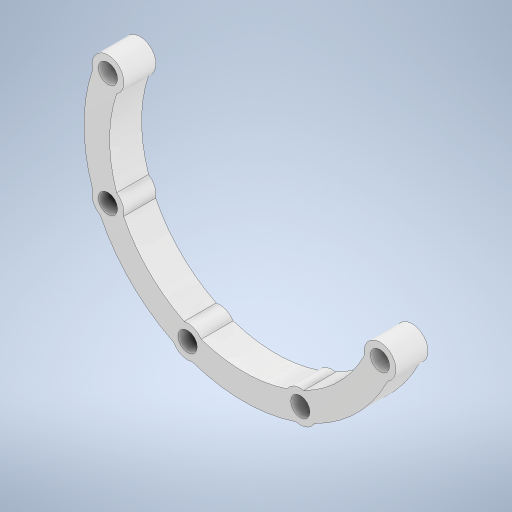
# Autodesk Inventor part: RP_Hip-Link-Limit-Long
Saved by Autodesk Inventor 2024.3 (Build 283343000, 343)
## iProperties
Created: 2025-01-05
Part Number: RP_Hip-Link-Limit-Long
Material: ABS プラスチック
Document SubType Name: Modeling
Designer: 佐藤智貴
Density: 1.06 g/cm^3
Appearance: 滑らか - 白
Mass: 12.4711 g
Surface Area: 64.1579 cm^2
Volume: 11.7652 cm^3
Author: 佐藤智貴
Autodesk Inventor part; units mm, degrees
ref_plane "YZ Plane" through (0, 0, 0) normal (1, 0, 0) x (0, 1, 0)
ref_plane "XZ Plane" through (0, 0, 0) normal (0, 1, 0) x (-1, 0, 0)
ref_plane "XY Plane" through (0, 0, 0) normal (0, 0, 1) x (1, 0, 0)
sketch "スケッチ1" plane through (0, 0, 0) normal (0, 0, 1) x (1, 0, 0)
  arc A0 (-41.8605, 19.0708) -> (-40.3368, 22.112) centre (0, 0) ccw
  line L0 (0, 0) -> (0, 54.8528)
  line L1 (0, 0) -> (-20.7697, 50.1426)
  circle A1 centre (-17.6034, 42.4985) radius 1.6
  circle A2 centre (-42.4985, 17.6034) radius 1.6
  circle A3 centre (-42.4985, -17.6034) radius 1.6
  circle A4 centre (-17.6034, -42.4985) radius 1.6
  circle A5 centre (17.6034, -42.4985) radius 1.6
  circle A6 centre (42.4985, -17.6034) radius 1.6
  circle A7 centre (42.4985, 17.6034) radius 1.6
  circle A8 centre (17.6034, 42.4985) radius 1.6
  line L2 (0, 0) -> (-55.1659, -46.2897)
  line L3 (-55.1659, -46.2897) -> (-55.1659, 46.2897)
  line L4 (-55.1659, 46.2897) -> (0, 0)
  line L5 (0, 0) -> (-76.7662, 0)
  circle A9 centre (-42.4985, 17.6034) radius 5
  circle A10 centre (-42.4985, -17.6034) radius 5
  circle A11 centre (-17.6034, -42.4985) radius 5
  circle A12 centre (17.6034, -42.4985) radius 5
  line L6 (0, 0) -> (55.1659, -46.2897)
  line L7 (55.1659, 46.2897) -> (0, 0)
  circle A13 centre (-17.6034, 42.4985) radius 5
  circle A14 centre (42.4985, -17.6034) radius 5
  arc A15 (-39.8089, 13.3884) -> (-39.8089, -13.3884) centre (0, 0) ccw
  arc A16 (-47.2999, 16.2085) -> (-47.2999, -16.2085) centre (0, 0) ccw
  arc A17 (-37.6162, -18.6821) -> (-18.6821, -37.6162) centre (0, 0) ccw
  arc A18 (-44.9073, -21.985) -> (-21.985, -44.9073) centre (0, 0) ccw
  arc A19 (-13.3884, -39.8089) -> (13.3884, -39.8089) centre (0, 0) ccw
  arc A20 (-16.2085, -47.2999) -> (16.2085, -47.2999) centre (0, 0) ccw
  arc A21 (18.6821, -37.6162) -> (37.6162, -18.6821) centre (0, 0) ccw
  arc A22 (39.8089, -13.3884) -> (-37.6162, 18.6821) centre (0, 0) ccw
  arc A23 (21.985, -44.9073) -> (44.9073, -21.985) centre (0, 0) ccw
  arc A24 (47.2999, -16.2085) -> (-44.9073, 21.985) centre (0, 0) ccw
  point P0 (-32.1739, 26.9971)
  point P1 (-38.3022, 32.1394)
  dimension "d0" = 92
  dimension "d3" = 22.5
  dimension "d4" = 3.2
  dimension "d7" = 360
  dimension "d9" = 80
  dimension "d10" = 40
  dimension "d18" = 10
  dimension "d19" = 10
  dimension "d20" = 10
  dimension "d21" = 10
  dimension "d24" = 10
  dimension "d25" = 10
  constraints: 44 point on circle, 24 centre point, 16 end point, 2 coincident, 2 symmetric about line, 2 vertical, 1 horizontal, 1 point on line, 20 other
  measures "d0" diameter of A0
  measures "d3" angle of L0 L1
  measures "d4" diameter of A1
  measures "d9" angle of L4 L2
  measures "d10" angle of L2 L5
  measures "d18" diameter of A9
  measures "d19" diameter of A10
  measures "d20" diameter of A11
  measures "d21" diameter of A12
  measures "d24" diameter of A14
  measures "d25" diameter of A13
extrude "押し出し1" add sketch "スケッチ1" along normal blind 10 contours A9 | A9 A15 L5 A0 | A0 L5 A16 A9 | L5 A15 A10 A0 | A0 A10 A16 L5 | A10 A0 A3 | A0 A3 A10 | A10 A0 L2 A18 | A17 A11 A0 L2 | L2 A0 A10 A17 | A21 A14 A0 L6 | L6 A0 A12 A21 | L2 A0 A11 A18 | A11 A0 A4 | L6 A23 A12 A0 | A0 A14 A23 L6 | A12 A0 A5 | A14 A0 A6 | A11 A0 A4 | A19 A12 A0 A11 | A12 A0 A5 | A0 A6 A14 | A11 A0 A12 A20
sketch "スケッチ2" plane through (0, 0, 10) normal (0, 0, 1) x (1, 0, 0)
  circle A0 centre (-42.4985, -17.6034) radius 1.6 projected
  circle A1 centre (-42.4985, -17.6034) radius 3
  circle A2 centre (-42.4985, 17.6034) radius 1.6 projected
  circle A3 centre (-42.4985, 17.6034) radius 3
  arc A4 (16.2085, -47.2999) -> (21.985, -44.9073) centre (17.6034, -42.4985) ccw projected
  arc A5 (-13.3884, -39.8089) -> (-18.6821, -37.6162) centre (-17.6034, -42.4985) ccw projected
  circle A6 centre (-17.6034, -42.4985) radius 3
  circle A7 centre (17.6034, -42.4985) radius 3
  arc A8 (44.9073, -21.985) -> (37.6162, -18.6821) centre (42.4985, -17.6034) ccw projected
  circle A9 centre (-17.6034, 42.4985) radius 1.6 projected
  circle A10 centre (-17.6034, 42.4985) radius 3
  circle A11 centre (42.4985, -17.6034) radius 3
  arc A12 (-37.6162, -18.6821) -> (-18.6821, -37.6162) centre (0, 0) ccw projected
  arc A13 (-37.6162, -18.6821) -> (-39.8089, -13.3884) centre (-42.4985, -17.6034) ccw projected
  arc A14 (-39.8089, 13.3884) -> (-39.8089, -13.3884) centre (0, 0) ccw projected
  arc A15 (-39.8089, 13.3884) -> (-47.2999, 16.2085) centre (-42.4985, 17.6034) ccw projected
  arc A16 (-47.2999, 16.2085) -> (-47.2999, -16.2085) centre (0, 0) ccw projected
  arc A17 (-47.2999, -16.2085) -> (-44.9073, -21.985) centre (-42.4985, -17.6034) ccw projected
  arc A18 (-44.9073, -21.985) -> (-21.985, -44.9073) centre (0, 0) ccw projected
  arc A19 (-21.985, -44.9073) -> (-16.2085, -47.2999) centre (-17.6034, -42.4985) ccw projected
  arc A20 (-16.2085, -47.2999) -> (16.2085, -47.2999) centre (0, 0) ccw projected
  arc A21 (21.985, -44.9073) -> (44.9073, -21.985) centre (0, 0) ccw projected
  arc A22 (18.6821, -37.6162) -> (37.6162, -18.6821) centre (0, 0) ccw projected
  arc A23 (18.6821, -37.6162) -> (13.3884, -39.8089) centre (17.6034, -42.4985) ccw projected
  arc A24 (-13.3884, -39.8089) -> (13.3884, -39.8089) centre (0, 0) ccw projected
  dimension "d14" = 6
  dimension "d15" = 6
  dimension "d22" = 6
  dimension "d23" = 6
  dimension "d26" = 6
  dimension "d27" = 6
  constraints: 6 centre point, 4 coincident
  measures "d14" diameter of A3
  measures "d15" diameter of A1
  measures "d22" diameter of A6
  measures "d23" diameter of A7
  measures "d26" diameter of A11
  measures "d27" diameter of A10
extrude "押し出し2" cut sketch "スケッチ2" against normal blind 5 contours A0 | A1 | A2 | A3 | A6 | A7 | A11
equation "\"d10\" = 0.5 * d9"
equation "\"d24\" = d21"
equation "\"d25\" = d18"
equation "\"d22\" = d15"
equation "\"d23\" = d15"
equation "\"d26\" = d23"
equation "\"d27\" = d14"
